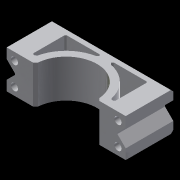
# Autodesk Inventor part: AXMM
Saved by Autodesk Inventor 2016 (Build 200138000, 138)
## iProperties
Created: 2017-07-16
Part Number: AXMM
Material: PC/ABS Plastic
Document SubType Name: Modeling
Designer: ludwi
Density: 0.357273 g/cm^3
Appearance: Smooth - White
Author: ludwi
Autodesk Inventor part; units mm, degrees
ref_plane "YZ Plane" through (0, 0, 0) normal (1, 0, 0) x (0, 1, 0)
ref_plane "XZ Plane" through (0, 0, 0) normal (0, 1, 0) x (-1, 0, 0)
ref_plane "XY Plane" through (0, 0, 0) normal (0, 0, 1) x (1, 0, 0)
sketch "Sketch1" plane through (0, 0, 0) normal (0, 0, 1) x (1, 0, 0)
  line L0 (0, 4) -> (100, 4) construction
  line L1 (0, 4) -> (0, 20) construction
  line L2 (12, 20) -> (0, 20) construction
  arc A0 (12, 20) -> (28, 20) centre (20, 20) ccw construction
  line L3 (38, 20) -> (28, 20) construction
  arc A1 (38, 20) -> (62, 20) centre (50, 20) ccw construction
  line L4 (72, 20) -> (62, 20) construction
  arc A2 (72, 20) -> (88, 20) centre (80, 20) ccw construction
  line L5 (100, 20) -> (88, 20) construction
  line L6 (100, 4) -> (100, 20) construction
  arc A3 (75.9, -36) -> (24.1, -36) centre (50, -36) ccw
  line L7 (100, 4) -> (0, 4)
  line L8 (100, 4) -> (0, 4)
  line L9 (0, 4) -> (0, -36)
  line L10 (100, -36) -> (100, 4)
  line L11 (100, -36) -> (75.9, -36)
  line L12 (24.1, -36) -> (0, -36)
  point P0 (0, 0)
  point P1 (50, 4)
  point P2 (50, -76)
  dimension "d0" = 51.8
  dimension "d1" = 40
  constraints: 12 end point, 4 equal length, 3 horizontal, 2 point on circle, 2 vertical alignment, 1 centre point, 1 horizontal alignment, 1 midpoint, 1 perpendicular
  measures "d0" diameter of A3
  measures "d1" distance of point (50, 4) A3.centre
extrude "Extrusion1" add sketch "Sketch1" against normal blind 32
sketch "Sketch2" plane through (0, -36, 0) normal (0, -1, 0) x (1, 0, 0)
  circle A0 centre (93.5, -25.5) radius 3
  circle A1 centre (93.5, -6.5) radius 3
  circle A2 centre (6.5, -25.5) radius 3
  circle A3 centre (6.5, -6.5) radius 3
  point P0 (0, 0)
  constraints: 4 centre point
extrude "Extrusion2" cut sketch "Sketch2" against normal through all
sketch "Sketch6" plane through (0, 0, 0) normal (0, 0, 1) x (1, 0, 0)
  line L0 (100, 4) -> (0, 4) construction
  line L1 (0, 4) -> (0, -36) construction
  line L2 (0, -36) -> (24.1, -36) construction
  arc A0 (75.9, -36) -> (24.1, -36) centre (50, -36) ccw construction
  line L3 (75.9, -36) -> (100, -36) construction
  line L4 (100, -36) -> (100, 4) construction
  line L5 (3.5, -36) -> (3.5, 4) construction
  line L6 (9.5, -36) -> (9.5, 4) construction
  line L7 (96.5, -36) -> (96.5, 4) construction
  line L8 (90.5, -36) -> (90.5, 4) construction
  line L9 (90.5, -36) -> (75.9, -36)
  arc A1 (75.9, -36) -> (24.1, -36) centre (50, -36) ccw
  line L10 (24.1, -36) -> (9.5, -36)
  line L11 (9.5, -36) -> (3.5, -36) projected
  line L12 (9.5, -36) -> (9.5, 4)
  line L13 (9.5, -36) -> (9.5, 4) projected
  line L14 (9.5, 4) -> (90.5, 4)
  line L15 (0, 4) -> (100, 4) projected
  line L16 (90.5, 4) -> (90.5, -36)
  line L17 (81.3307, -30) -> (84.5, -30)
  line L18 (84.5, -30) -> (84.5, -2)
  line L19 (84.5, -2) -> (15.5, -2)
  line L20 (15.5, -2) -> (15.5, -30)
  line L21 (15.5, -30) -> (18.6693, -30)
  line L22 (55, -2) -> (55, -4.4943)
  line L23 (45, -4.4943) -> (45, -2)
  arc A2 (81.3307, -30) -> (55, -4.4943) centre (50, -36) ccw
  arc A3 (45, -4.4943) -> (18.6693, -30) centre (50, -36) ccw
  point P0 (0, 0)
  point P1 (50, -0.8369)
  point P2 (50, -2)
  dimension "d39" = 6
  constraints: 24 end point, 6 collinear, 6 point on circle, 3 centre point, 2 point on line, 1 concentric, 1 midpoint, 1 parallel, 1 vertical alignment, 4 other
  measures "d39" distance between parallel lines of L8 L18
extrude "Extrusion6" cut sketch "Sketch6" against normal through all contours A2 L22 L19 L18 L17 | L23 A3 L21 L20 L19
chamfer "Chamfer2" distance 2 angle 45 4 edges at (50, 4, 0) (50, 4, -32) (75.9, -36, -16) (24.1, -36, -16)
sketch "Sketch8" plane through (0, -36, -32) normal (0, -1, 0) x (1, 0, 0)
  line L0 (0, 32) -> (22.1, 32) construction
  line L1 (0, 32) -> (0, 0) construction
  line L2 (22.1, 0) -> (0, 0) construction
  circle A0 centre (6.5, 25.5) radius 3 construction
  circle A1 centre (6.5, 6.5) radius 3 construction
  line L3 (100, 0) -> (77.9, 0) construction
  line L4 (100, 32) -> (100, 0) construction
  line L5 (77.9, 32) -> (100, 32) construction
  circle A2 centre (93.5, 25.5) radius 3 construction
  circle A3 centre (93.5, 6.5) radius 3 construction
  line L6 (13.5, 0) -> (13.5, 32) construction
  line L7 (88, 0) -> (88, 32) construction
  line L8 (12, 32) -> (12, 0) construction
  line L9 (86.5, 32) -> (86.5, 0) construction
  line L10 (100, 32) -> (100, 0) projected
  line L11 (100, 8.5) -> (93, 15.5)
  line L12 (93, 15.5) -> (93, 16.5)
  line L13 (93, 16.5) -> (100, 23.5)
  line L14 (100, 23.5) -> (100, 8.5)
  line L15 (75.8228, 0) -> (24.1772, 0) construction
  line L16 (24.1772, 32) -> (75.8228, 32) construction
  line L17 (75.8228, 0) -> (24.1772, 0) construction
  line L18 (50, 0) -> (50, 32) construction
  line L19 (0, 8.5) -> (7, 15.5)
  line L20 (7, 15.5) -> (7, 16.5)
  line L21 (7, 16.5) -> (0, 23.5)
  line L22 (0, 23.5) -> (0, 8.5)
  line L23 (24.1772, 0) -> (24.1772, 32) projected
  line L24 (75.8228, 32) -> (75.8228, 0) projected
  line L25 (77.9, 0) -> (77.9, 32) projected
  line L26 (22.1, 32) -> (22.1, 0) projected
  point P0 (0, 32)
  point P1 (100, 30)
  point P2 (100, 2)
  point P3 (93, 16)
  point P4 (100, 16)
  point P5 (100, 16)
  point P6 (7, 16)
  point P7 (24.1, 0)
  point P8 (75.9, 0)
  dimension "d34" = 7
  dimension "d35" = 15
  dimension "d36" = 45
  constraints: 18 end point, 5 midpoint, 5 symmetric about line, 2 horizontal alignment, 2 parallel, 2 point on line
  measures "d34" distance between parallel lines of L10 L12
  measures "d35" distance of L13.end L11.start
  measures "d36" angle of L4 L11
extrude "Extrusion8" cut sketch "Sketch8" against normal through all
chamfer "Chamfer4" distance 1 angle 45 10 edges at (18.6693, -30, -16) (15.5, -30, -16) (15.5, -2, -16) (45, -2, -16) (45, -4.4943, -16) (55, -2, -16) (55, -4.4943, -16) (84.5, -2, -16) (84.5, -30, -16) (81.3307, -30, -16)
body "Solid1"
